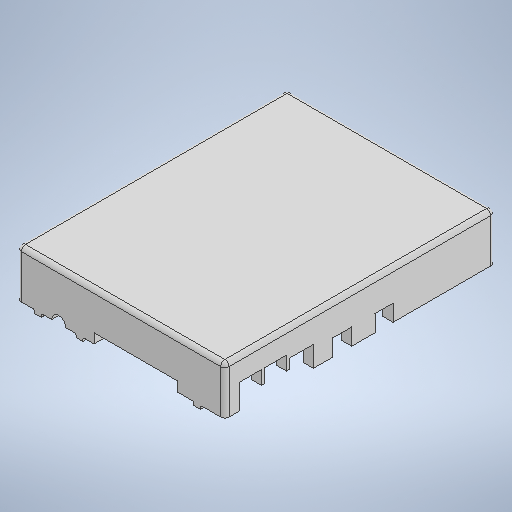
# Autodesk Inventor part: Electronic Lid - Final
Saved by Autodesk Inventor 2025.2 (Build 292293000, 293)
## iProperties
Created: 2025-03-21
Part Number: Electronic Lid - Final
Material: Generic
Document SubType Name: Modeling
Designer: caomi
Density: 1 g/cm^3
Appearance: Default
Author: caomi
Autodesk Inventor part; units mm, degrees
ref_plane "YZ Plane" through (0, 0, 0) normal (1, 0, 0) x (0, 1, 0)
ref_plane "XZ Plane" through (0, 0, 0) normal (0, 1, 0) x (-1, 0, 0)
ref_plane "XY Plane" through (0, 0, 0) normal (0, 0, 1) x (1, 0, 0)
sketch "Sketch1" plane through (0, 0, 0) normal (0, 1, 0) x (-1, 0, 0)
  line L0 (0, 0) -> (-135, 0)
  line L1 (-135, 0) -> (-135, 180)
  line L2 (-135, 180) -> (0, 180)
  line L3 (0, 180) -> (0, 0)
  dimension "d9" = 135
  dimension "d21" = 180
  constraints: 8 end point, 2 parallel, 1 horizontal, 1 perpendicular
  measures "d9" distance of L1.end L2.end
  measures "d21" distance of L2.end L0.start
extrude "Extrusion1" add sketch "Sketch1" along normal blind 27
shell "Shell1" thickness 7.5 outward yes removed faces 1 at (90, 0, 60)
sketch "Sketch2" plane through (0, 0, 0) normal (0, -1, 0) x (1, 0, 0)
  line L0 (142.5, 187.5) -> (142.5, -7.5) projected
  line L1 (142.5, 177) -> (135, 177)
  line L2 (135, 177) -> (135, 161)
  line L3 (135, 161) -> (142.5, 161)
  line L4 (142.5, 161) -> (142.5, 177)
  line L5 (142.5, 159) -> (135, 159)
  line L6 (135, 159) -> (135, 143)
  line L7 (135, 143) -> (142.5, 143)
  line L8 (142.5, 143) -> (142.5, 159)
  line L9 (0, 180) -> (135, 180) projected
  line L10 (142.5, 141) -> (135, 141)
  line L11 (135, 141) -> (135, 123.5)
  line L12 (135, 123.5) -> (142.5, 123.5)
  line L13 (142.5, 123.5) -> (142.5, 141)
  line L14 (135, 180) -> (135, 0) projected
  line L15 (142.5, 109.5) -> (135, 109.5)
  line L16 (135, 109.5) -> (135, 95.86)
  line L17 (135, 95.86) -> (142.5, 95.86)
  line L18 (142.5, 95.86) -> (142.5, 109.5)
  line L19 (142.5, 79) -> (135, 79)
  line L20 (135, 79) -> (135, 66)
  line L21 (135, 66) -> (142.5, 66)
  line L22 (142.5, 66) -> (142.5, 79)
  line L23 (-7.5, 187.5) -> (142.5, 187.5) projected
  line L24 (108, 187.5) -> (48, 187.5)
  line L25 (48, 187.5) -> (48, 180)
  line L26 (48, 180) -> (108, 180)
  line L27 (108, 180) -> (108, 187.5)
  point P0 (138.75, 161)
  point P1 (142.5, 66)
  point P2 (135, 79)
  point P3 (142.5, 95.86)
  point P4 (135, 109.5)
  point P5 (142.5, 123.5)
  point P6 (142.5, 161)
  point P7 (108, 180)
  point P8 (48, 187.5)
  dimension "d10" = 3
  dimension "d12" = 21
  dimension "d16" = 70.5
  dimension "d18" = 101
  dimension "d19" = 13
  dimension "d20" = 13.64
  dimension "d22" = 27
  dimension "d23" = 87
  dimension "d27" = 19
  dimension "d28" = 37
  dimension "d29" = 39
  dimension "d30" = 56.5
  constraints: 48 end point, 12 parallel, 12 point on line, 6 horizontal, 6 perpendicular, 1 midpoint
  measures "d10" distance between parallel lines of L1 L9
  measures "d12" distance from line of L5 L9.end
  measures "d16" distance of L9.end L15.end
  measures "d18" distance from line of L9.end L19
  measures "d19" distance of L21.end L19.start
  measures "d20" distance of L17.end L15.start
  measures "d22" distance of L9.end L26.end
  measures "d23" distance of L9.end L25.end
  measures "d27" distance from line of L9.end L3
  measures "d28" vertical distance of L9.end L7.end
  measures "d29" vertical distance of L9.end L10.start
  measures "d30" vertical distance of L9.end L12.end
extrude "Board Ports" cut sketch "Sketch2" against normal blind 18 contours L0 L3 L2 L1 | L0 L7 L6 L5
extrude "Extrusion9" cut sketch "Sketch2" against normal blind 7 contours L27 L9 L25 L23
extrude "Extrusion10" cut sketch "Sketch2" against normal blind 8 contours L0 L5 L14 L3 | L0 L10 L14 L7
extrude "Extrusion11" cut sketch "Sketch2" against normal blind 15 contours L0 L12 L11 L10
extrude "Extrusion12" cut sketch "Sketch2" against normal blind 12 contours L0 L17 L14 L15 | L0 L21 L14 L19
fillet "Fillet1" radius 3 8 edges at (142.5, 17.25, 187.5) (-7.5, 17.25, 187.5) (142.5, 17.25, -7.5) (-7.5, 17.25, -7.5) (-7.5, 34.5, 90) (67.5, 34.5, -7.5) (67.5, 34.5, 187.5) (142.5, 34.5, 90)
ref_plane "Work Plane6" through (122.5, 0, 177) normal (1, 0, 0) x (0, 0, -1)
ref_plane "Work Plane7" through (37.5, 0, 177) normal (1, 0, 0) x (0, 0, -1)
ref_plane "Work Plane8" through (12.5, 0, 177) normal (1, 0, 0) x (0, 0, -1)
ref_plane "Work Plane9" through (7.5, 0, 177) normal (1, 0, 0) x (0, 0, -1)
sketch "Sketch3" plane through (142.5, 0, 95.86) normal (1, 0, 0) x (0, 0, -1)
  line L0 (-91.64, 31.5) -> (-91.64, 0) projected
  line L1 (-91.64, 0) -> (-90.14, 0)
  line L2 (-90.14, 0) -> (-90.14, -2.5)
  line L3 (-90.14, -2.5) -> (-91.64, -2.5)
  line L4 (-91.64, -2.5) -> (-91.64, 0)
  line L5 (-90.14, -2.5) -> (-89.14, -1.5)
  line L6 (-89.14, -1.5) -> (-90.14, -0.5)
  line L7 (-89.14, -1.5) -> (-90.14, -1.5) construction
  line L8 (-88.64, 31.5) -> (100.36, 31.5) projected
  line L9 (5.86, 51.3756) -> (5.86, -39.6704) construction
  line L10 (103.36, 0) -> (101.86, 0)
  line L11 (101.86, 0) -> (101.86, -2.5)
  line L12 (101.86, -2.5) -> (103.36, -2.5)
  line L13 (103.36, -2.5) -> (103.36, 0)
  line L14 (101.86, -2.5) -> (100.86, -1.5)
  line L15 (100.86, -1.5) -> (101.86, -0.5)
  line L16 (100.86, -1.5) -> (101.86, -1.5) construction
  line L17 (100.36, 31.5) -> (100.36, 0) projected
  line L18 (-88.64, 0) -> (-88.64, 31.5) projected
  line L19 (-88.64, 0) -> (-81.14, 0) projected
  line L20 (-81.14, 0) -> (-81.14, 18) projected
  line L21 (-81.14, 18) -> (-65.14, 18) projected
  line L22 (-65.14, 18) -> (-65.14, 8) projected
  line L23 (-65.14, 8) -> (-63.14, 8) projected
  line L24 (-63.14, 8) -> (-63.14, 18) projected
  line L25 (-63.14, 18) -> (-47.14, 18) projected
  line L26 (-47.14, 18) -> (-47.14, 8) projected
  line L27 (-47.14, 8) -> (-45.14, 8) projected
  line L28 (-45.14, 8) -> (-45.14, 15) projected
  line L29 (-45.14, 15) -> (-27.64, 15) projected
  line L30 (-27.64, 15) -> (-27.64, 0) projected
  line L31 (-27.64, 0) -> (-13.64, 0) projected
  line L32 (-13.64, 0) -> (-13.64, 12) projected
  line L33 (-13.64, 12) -> (0, 12) projected
  line L34 (0, 12) -> (0, 0) projected
  line L35 (0, 0) -> (16.86, 0) projected
  line L36 (16.86, 0) -> (16.86, 12) projected
  line L37 (16.86, 12) -> (29.86, 12) projected
  line L38 (29.86, 12) -> (29.86, 0) projected
  line L39 (29.86, 0) -> (100.36, 0) projected
  point P0 (95.86, 0)
  point P1 (5.86, 31.5)
  dimension "d35" = 1.5
  dimension "d36" = 2.5
  dimension "d37" = 1
  dimension "d38" = 45
  constraints: 30 end point, 7 symmetric about line, 5 point on line, 2 parallel, 2 perpendicular, 1 horizontal, 1 midpoint, 1 vertical, 1 other
  measures "d35" distance of L2.end L3.end
  measures "d36" distance of L3.end L0.end
  measures "d37" distance of L5.end L7.end
  measures "d38" angle of L2 L5
extrude "Extrusion3" add sketch "Sketch3" along normal mid plane 5 from surface at -20 contours L1 L2 L3 L4 | L6 L5 L2
extrude "Extrusion8" add sketch "Sketch3" along normal mid plane 5 from surface at -105 contours L1 L2 L3 L4 | L6 L5 L2
extrude "Extrusion5" add sketch "Sketch3" along normal mid plane 5 from surface at -135 contours L1 L2 L3 L4 | L6 L5 L2
extrude "Extrusion6" add sketch "Sketch3" along normal mid plane 5 from surface at -20 contours L13 L12 L11 L10 | L11 L14 L15
extrude "Extrusion7" add sketch "Sketch3" along normal mid plane 5 from surface at -130 contours L13 L12 L11 L10 | L11 L14 L15
sketch "Sketch4" plane through (48, 7, 187.5) normal (0, 0, 1) x (1, 0, 0)
  line L0 (-38, -7) -> (-13, -7) projected
  circle A0 centre (-25.5, -7) radius 5
  line L1 (-55.5, 24.5) -> (-55.5, -7) projected
  point P0 (-48, -7)
  dimension "d64" = 30
  dimension "d67" = 10
  constraints: 1 centre point, 1 midpoint
  measures "d64" distance from line of L1 A0.centre
  measures "d67" diameter of A0
extrude "Extrusion13" cut sketch "Sketch4" against normal up to surface (7.5 mm away)
ref_plane "Work Plane10" through (0, 0, 180) normal (0, -1, 0) x (1, 0, 0)
sketch "Sketch5" plane through (0, 0, 180) normal (0, -1, 0) x (1, 0, 0)
  line L0 (27.75, 1.5) -> (17.25, 1.5)
  line L1 (17.25, 1.5) -> (15.5, -11.5)
  line L2 (15.5, -11.5) -> (29.5, -11.5)
  line L3 (29.5, -11.5) -> (27.75, 1.5)
  line L4 (22.5, 3.5405) -> (22.5, -12.0447) construction
  line L5 (17.5, 7.5) -> (27.5, 7.5) projected
  line L6 (-7.5, -184.5) -> (-7.5, 4.5) projected
  point P0 (0, -180)
  dimension "d69" = 10.5
  dimension "d70" = 14
  dimension "d71" = 13
  dimension "d72" = 6
  dimension "d73" = 30
  constraints: 10 end point, 2 horizontal, 1 vertical, 1 other
  measures "d69" distance of L0.start L0.end
  measures "d70" distance of L1.end L2.end
  measures "d71" distance between parallel lines of L2 L0
  measures "d72" distance between parallel lines of L5 L0
  measures "d73" distance between parallel lines of L6 L4
extrude "Extrusion14" cut sketch "Sketch5" against normal blind 3
sketch "Sketch6" plane through (0, 0, 0) normal (1, 0, 0) x (0, 0, -1)
  line L0 (0, 0) -> (-180, 0) projected
  line L1 (0, 0) -> (0, 27) projected
  circle A0 centre (-90, 9) radius 11.25
  point P0 (-83.25, 0)
  point P1 (-96.75, 0)
  dimension "d76" = 9
  dimension "d77" = 90
  dimension "d78" = 22.5
  constraints: 1 centre point
  measures "d76" distance from line of L0 A0.centre
  measures "d77" distance from line of L1 A0.centre
  measures "d78" diameter of A0
extrude "Extrusion15" cut sketch "Sketch6" against normal through all contours L0 A0 picked at (-87.8593, 7.2825)
fillet "Fillet2" radius 1 5 edges at (122.5, -1.5, 185) (37.5, -1.5, 185) (7.5, -1.5, 185) (122.5, -1.5, -5) (12.5, -1.5, -5)
fillet "Fillet3" radius 1 10 edges at (125, 0, -6.75) (120, 0, -6.75) (15, 0, -6.75) (10, 0, -6.75) (5, 0, 186.75) (10, 0, 186.75) (35, 0, 186.75) (40, 0, 186.75) (120, 0, 186.75) (125, 0, 186.75)
body "Solid1"
